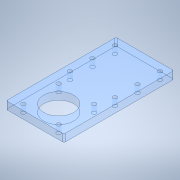
# Autodesk Inventor part: afirma_motor_lado
Saved by Autodesk Inventor 2022 (Build 260153000, 153)
## iProperties
Created: 2022-05-04
Part Number: afirma_motor_lado
Material: Generic
Document SubType Name: Modeling
Designer: ferna
Density: 1 g/cm^3
Appearance: Blue - Glazing
Author: ferna
Autodesk Inventor part; units mm, degrees
ref_plane "YZ Plane" through (0, 0, 0) normal (1, 0, 0) x (0, 1, 0)
ref_plane "XZ Plane" through (0, 0, 0) normal (0, 1, 0) x (-1, 0, 0)
ref_plane "XY Plane" through (0, 0, 0) normal (0, 0, 1) x (1, 0, 0)
sketch "Sketch1" plane through (0, 0, 0) normal (0, 1, 0) x (-1, 0, 0)
  arc A0 (-15, 27) -> (-13, 25) centre (-13, 27) ccw
  line L0 (-15, 27) -> (-15, 53)
  arc A1 (-13, 55) -> (-15, 53) centre (-13, 53) ccw
  line L1 (-13, 55) -> (13, 55)
  arc A2 (15, 53) -> (13, 55) centre (13, 53) ccw
  line L2 (15, 53) -> (15, 27)
  arc A3 (13, 25) -> (15, 27) centre (13, 27) ccw
  line L3 (13, 25) -> (-13, 25)
  arc A4 (36.5, 1.5) -> (38.5, 3.5) centre (36.5, 3.5) ccw
  line L4 (38.5, 3.5) -> (38.5, 76.5)
  arc A5 (38.5, 76.5) -> (36.5, 78.5) centre (36.5, 76.5) ccw
  line L5 (36.5, 78.5) -> (-36.5, 78.5)
  arc A6 (-36.5, 78.5) -> (-38.5, 76.5) centre (-36.5, 76.5) ccw
  line L6 (-38.5, 76.5) -> (-38.5, 3.5)
  arc A7 (-38.5, 3.5) -> (-36.5, 1.5) centre (-36.5, 3.5) ccw
  line L7 (-36.5, 1.5) -> (36.5, 1.5)
  circle A8 centre (0, 60) radius 2.5
  circle A9 centre (-10, 70) radius 2.5
  circle A10 centre (10, 70) radius 2.5
  circle A11 centre (30, 70) radius 2.75
  circle A12 centre (10, 10) radius 2.5
  circle A13 centre (30, 10) radius 2.75
  circle A14 centre (0, 20) radius 2.5
  circle A15 centre (20, 30) radius 2.5
  circle A16 centre (20, 60) radius 2.5
  circle A17 centre (20, 50) radius 2.5
  circle A18 centre (-20, 30) radius 2.5
  circle A19 centre (-30, 40) radius 2.75
  circle A20 centre (-20, 20) radius 2.5
  circle A21 centre (20, 20) radius 2.5
  circle A22 centre (-20, 60) radius 2.5
  circle A23 centre (-10, 10) radius 2.5
  circle A24 centre (-30, 10) radius 2.75
  circle A25 centre (-30, 70) radius 2.75
  circle A26 centre (30, 40) radius 2.75
  circle A27 centre (-20, 50) radius 2.5
  line L8 (13, 53) -> (-13, 27)
  line L9 (-13, 53) -> (13, 27)
  line L10 (0, 0) -> (0, 40)
  line L11 (0, 0) -> (0, -40)
  line L12 (36.4941, 78.5) -> (-36.5, 78.5)
  line L13 (-38.5, 78.5) -> (-38.5, -56.3967)
  line L14 (-36.5, -66.5) -> (36.4941, -66.5)
  line L15 (38.4941, -59.5) -> (38.4941, 76.5)
  arc A28 (38.4941, 76.5) -> (36.4941, 78.5) centre (36.4941, 76.5) ccw
  arc A29 (-36.5, 78.5) -> (-38.5, 76.5) centre (-36.5, 76.5) ccw
  arc A30 (-38.5, -56.3967) -> (-36.5, -58.3967) centre (-36.5, -56.3967) ccw
  arc A31 (36.4941, -66.5) -> (38.4941, -64.5) centre (36.4941, -64.5) ccw
  line L16 (-38.5, -59.5) -> (-38.5, -56.3967)
  arc A32 (-38.5, -64.5) -> (-36.5, -66.5) centre (-36.5, -64.5) ccw
  circle A33 centre (0, -35) radius 20
  arc A34 (-25.4017, -7.1967) -> (-28.4017, -10.1967) centre (-25.4017, -10.1967) ccw
  line L17 (-28.4017, -10.1967) -> (-28.4017, -61.3967)
  arc A35 (-28.4017, -61.3967) -> (-26.4017, -63.3967) centre (-26.4017, -61.3967) ccw
  line L18 (-26.4017, -63.3967) -> (24.7983, -63.3967)
  arc A36 (24.7983, -63.3967) -> (27.7983, -60.3967) centre (24.7983, -60.3967) ccw
  line L19 (27.7983, -60.3967) -> (27.7983, -10.1967)
  arc A37 (27.7983, -10.1967) -> (24.7983, -7.1967) centre (24.7983, -10.1967) ccw
  line L20 (24.7983, -7.1967) -> (-25.4017, -7.1967)
  circle A38 centre (23.2983, -11.6967) radius 2.75
  circle A39 centre (-23.9017, -11.6967) radius 2.75
  circle A40 centre (23.2983, -58.8967) radius 2.75
  circle A41 centre (-23.9017, -58.8967) radius 2.75
  line L21 (38.4941, -59.5) -> (38.4941, -64.5)
  line L22 (-38.5, -64.5) -> (-38.5, -59.5)
  line L23 (-10, 40) -> (11.2302, 40)
  line L24 (0, 80) -> (0, 40)
  line L25 (0, 80) -> (0, 120)
  line L26 (-38.5, 1.5) -> (-38.5, 136.3967)
  line L27 (-36.5, 146.5) -> (36.4941, 146.5)
  line L28 (38.4941, 139.5) -> (38.4941, 3.5)
  arc A42 (-36.5, 138.3967) -> (-38.5, 136.3967) centre (-36.5, 136.3967) ccw
  arc A43 (38.4941, 144.5) -> (36.4941, 146.5) centre (36.4941, 144.5) ccw
  line L29 (-38.5, 139.5) -> (-38.5, 136.3967)
  arc A44 (-36.5, 146.5) -> (-38.5, 144.5) centre (-36.5, 144.5) ccw
  circle A45 centre (0, 115) radius 20
  arc A46 (-28.4017, 90.1967) -> (-25.4017, 87.1967) centre (-25.4017, 90.1967) ccw
  line L30 (-28.4017, 90.1967) -> (-28.4017, 141.3967)
  arc A47 (-26.4017, 143.3967) -> (-28.4017, 141.3967) centre (-26.4017, 141.3967) ccw
  line L31 (-26.4017, 143.3967) -> (24.7983, 143.3967)
  arc A48 (27.7983, 140.3967) -> (24.7983, 143.3967) centre (24.7983, 140.3967) ccw
  line L32 (27.7983, 140.3967) -> (27.7983, 90.1967)
  arc A49 (24.7983, 87.1967) -> (27.7983, 90.1967) centre (24.7983, 90.1967) ccw
  line L33 (24.7983, 87.1967) -> (-25.4017, 87.1967)
  circle A50 centre (23.2983, 91.6967) radius 2.75
  circle A51 centre (-23.9017, 91.6967) radius 2.75
  circle A52 centre (23.2983, 138.8967) radius 2.75
  circle A53 centre (-23.9017, 138.8967) radius 2.75
  line L34 (38.4941, 139.5) -> (38.4941, 144.5)
  line L35 (-38.5, 144.5) -> (-38.5, 139.5)
  point P0 (-38.5, 1.5)
  point P1 (0, 40)
  point P2 (-38.5, -61.5)
  point P3 (36.4941, 78.5)
  point P4 (38.4941, 3.3463)
  point P5 (36.5, 78.5)
  point P6 (0, 1.5)
  point P7 (36.4941, 78.5)
  point P8 (36.4941, -66.5)
  point P9 (-38.5, 141.5)
  point P10 (38.4941, 76.6537)
  point P11 (36.4941, 146.5)
  dimension "d0" = 40
  dimension "d1" = 40
  dimension "d2" = 2
  dimension "d5" = 145
  dimension "d6" = 0
  dimension "d7" = 2
  dimension "d13" = 5.5
  dimension "d14" = 5.5
  dimension "d15" = 5.5
  dimension "d16" = 5.5
  dimension "d17" = 5.5
  dimension "d18" = 5.5
  dimension "d20" = 40
  dimension "d21" = 5.5
  dimension "d22" = 5.5
  dimension "d23" = 5.5
  dimension "d24" = 5.5
  constraints: 72 end point, 54 centre point, 48 point on circle, 35 symmetric about line, 6 point on line, 6 tangent, 4 vertical, 3 equal radius, 3 parallel, 2 horizontal, 1 midpoint, 1 perpendicular, 12 other
  measures "d0" distance of L10.start L10.end
  measures "d1" distance of L10.start L11.end
  measures "d2" radius of A28
  measures "d5" distance between parallel lines of L12 L14
  measures "d6" distance between parallel lines of L5 L12
  measures "d7" radius of A32
  measures "d13" diameter of A11
  measures "d14" diameter of A26
  measures "d15" diameter of A13
  measures "d16" diameter of A25
  measures "d17" diameter of A19
  measures "d18" diameter of A24
  measures "d20" diameter of A33
  measures "d21" diameter of A38
  measures "d22" diameter of A39
  measures "d23" diameter of A41
  measures "d24" diameter of A40
extrude "Extrusion1" add sketch "Sketch1" along normal blind 10 contours A0 L3 L10 A14 L7 A7 L6 A6 L5 L24 A8 L1 A1 L0 | L3 A3 L2 A2 L1 L24 A8 L5 A28 L15 A4 L7 L10 A14 | L10 A14 | A14 L10 | L24 A8 | A8 L24 | L7 A4 L15 L21 A31 L14 A32 L22 L16 L13 A7 | L20 A37 L19 A36 L18 A35 L17 A34 | L5 A6 L13 L26 L29 L35 A44 L27 A43 L34 L28 A5 | L33 A46 L30 A47 L31 A48 L32 A49 | A9 | A10 | A12 | A15 | A16 | A17 | A18 | A20 | A21 | A22 | A23 | A27
sketch "Sketch3" plane through (0, 10, 0) normal (0, 1, 0) x (1, 0, 0)
  line L0 (15, -27) -> (15, -53) projected
  arc A0 (15, -27) -> (13, -25) centre (13, -27) ccw projected
  line L1 (-13, -25) -> (13, -25) projected
  arc A1 (-13, -25) -> (-15, -27) centre (-13, -27) ccw projected
  line L2 (-15, -53) -> (-15, -27) projected
  line L3 (13, -55) -> (-13, -55) projected
  arc A2 (13, -55) -> (15, -53) centre (13, -53) ccw projected
  arc A3 (-15, -53) -> (-13, -55) centre (-13, -53) ccw projected
  point P0 (0, 0)
extrude "Extrusion2" add sketch "Sketch3" against normal blind 10
sketch "Sketch5" plane through (0, 10, 0) normal (0, 1, 0) x (1, 0, 0)
  circle A0 centre (-23.2983, 11.6967) radius 2.75
  line L0 (8.6601, 21.3463) -> (-11.3399, 21.3463)
  line L1 (8.6601, 51.3463) -> (8.6601, 21.3463)
  line L2 (8.6601, 21.3463) -> (-11.3399, 21.3463)
  arc A1 (-21.3399, 31.3463) -> (-11.3399, 21.3463) centre (-11.3399, 31.3463) ccw
  line L3 (-21.3399, 31.3463) -> (-21.3399, 41.3463)
  arc A2 (-11.3399, 51.3463) -> (-21.3399, 41.3463) centre (-11.3399, 41.3463) ccw
  line L4 (-11.3399, 51.3463) -> (8.6601, 51.3463)
  circle A3 centre (23.9017, 11.6967) radius 2.75
  circle A4 centre (23.9017, 58.8967) radius 2.75
  circle A5 centre (-23.2983, 11.6967) radius 2.75
  circle A6 centre (-23.2983, 58.8967) radius 2.75
  line L5 (37.0974, 65.5992) -> (-35.8967, 65.5992)
  arc A7 (-35.8967, 65.5992) -> (-37.8967, 63.5992) centre (-35.8967, 63.5992) ccw
  line L6 (-37.8967, 63.5992) -> (-37.8967, 6.0933)
  line L7 (-37.8967, 6.0933) -> (-37.8967, 3.0933)
  line L8 (39.0974, 3.0933) -> (-37.8967, 3.0933)
  line L9 (39.0974, 63.5992) -> (39.0974, 3.0933)
  arc A8 (39.0974, 63.5992) -> (37.0974, 65.5992) centre (37.0974, 63.5992) ccw
  circle A9 centre (-23.2983, 11.6967) radius 2.75 projected
  point P0 (0, 0)
  point P1 (0.6033, 35.5933)
  point P2 (-11.3399, 21.3463)
  constraints: 20 end point, 9 centre point, 8 point on circle
sketch "Sketch6" plane through (0, 10, 0) normal (0, 1, 0) x (1, 0, 0)
  circle A0 centre (0, 35) radius 20 projected
  point P0 (0, 0)
extrude "Extrusion3" add sketch "Sketch6" against normal up to surface (10 mm away)
extrude "Extrusion4" cut sketch "Sketch5" against normal blind 10 contours L0 A1 L3 A2 L4 L1
sketch "Sketch7" plane through (-38.4941, 0, 76.6537) normal (-1, 0, 0) x (0, 0, 1)
  line L0 (67.8463, 10) -> (-141.1537, 10) projected
  line L1 (67.8463, 0) -> (-141.1537, 0) projected
  line L2 (2.4973, 10) -> (-2.5509, 10)
  line L3 (-2.5509, 10) -> (-2.5509, 0)
  line L4 (-2.5509, 0) -> (2.4973, 0)
  line L5 (2.4973, 0) -> (2.4973, 10)
  point P0 (-76.6537, 0)
  constraints: 8 end point, 2 parallel, 2 point on line, 1 horizontal, 1 perpendicular
extrude "Extrusion5" add sketch "Sketch7" against normal blind 4
sketch "Sketch8" plane through (0, 10, 0) normal (0, 1, 0) x (1, 0, 0)
  line L0 (-38.4941, 64.5) -> (-38.4941, -144.5) projected
  line L1 (-38.4941, 0) -> (43.0425, 0)
  line L2 (43.0425, 0) -> (43.0425, 71.8354)
  line L3 (43.0425, 71.8354) -> (-38.4941, 71.8354)
  line L4 (-38.4941, 71.8354) -> (-38.4941, 0)
  point P0 (0, 0)
  constraints: 8 end point, 2 parallel, 1 horizontal, 1 perpendicular, 1 point on line
extrude "Extrusion6" cut sketch "Sketch8" against normal through all
fillet "Fillet1" radius 2 2 edges at (38.5, 5, 0) (-38.4941, 5, 0)
body "Solid1"
